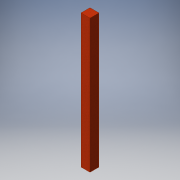
# Autodesk Inventor part: Front Post North Side
Saved by Autodesk Inventor 2016 (Build 200138000, 138)
## iProperties
Created: 2015-05-30
Part Number: Front Post North Side
Material: Wood (Oak)
Document SubType Name: Modeling
Designer: steele
Density: 0.76 g/cm^3
Appearance: White Oak - Natural Medium Gloss
Author: steele
Autodesk Inventor part; units mm, degrees
ref_plane "YZ Plane" through (0, 0, 0) normal (1, 0, 0) x (0, 1, 0)
ref_plane "XZ Plane" through (0, 0, 0) normal (0, 1, 0) x (-1, 0, 0)
ref_plane "XY Plane" through (0, 0, 0) normal (0, 0, 1) x (1, 0, 0)
sketch "Sketch1" plane through (0, 0, 0) normal (0, 1, 0) x (-1, 0, 0)
  line L0 (-44.45, 44.45) -> (-44.45, -44.45)
  line L1 (-44.45, -44.45) -> (44.45, -44.45)
  line L2 (44.45, -44.45) -> (44.45, 44.45)
  line L3 (44.45, 44.45) -> (-44.45, 44.45)
  line L4 (-44.45, 44.45) -> (44.45, -44.45) construction
  line L5 (-44.45, -44.45) -> (44.45, 44.45) construction
  point P0 (0, 0)
  dimension "d0" = 88.9
  constraints: 12 end point, 2 midpoint, 2 parallel, 2 perpendicular, 1 vertical
  measures "d0" distance of L0.start L0.end
extrude "Extrusion1" add sketch "Sketch1" along normal blind 1327.15
body "Solid1"
